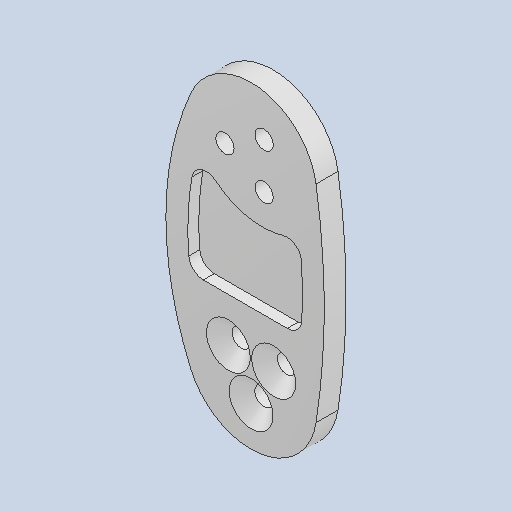
# Autodesk Inventor part: クランク_中間
Saved by Autodesk Inventor 2023 (Build 270158000, 158)
## iProperties
Created: 2022-01-08
Part Number: クランク_中間
Material: Aluminum 2014-T6
Document SubType Name: Modeling
Designer: acps
Density: 2.78927 g/cm^3
Appearance: Satin
Author: acps
Autodesk Inventor part; units mm, degrees
ref_plane "YZ Plane" through (0, 0, 0) normal (1, 0, 0) x (0, 1, 0)
ref_plane "XZ Plane" through (0, 0, 0) normal (0, 1, 0) x (-1, 0, 0)
ref_plane "XY Plane" through (0, 0, 0) normal (0, 0, 1) x (1, 0, 0)
sketch "Sketch2" plane through (0, 0, 0) normal (0, 0, 1) x (1, 0, 0)
  line L0 (-3.5796, 0) -> (-32.4095, 0) construction
  line L1 (-3.5796, 0) -> (-16.3075, 12.7279) construction
  line L2 (-3.5796, 0) -> (-16.3075, -12.7279) construction
  line L3 (-16.3075, 12.7279) -> (-16.3075, -12.7279) construction
  circle A0 centre (-14.5177, 15.8279) radius 1.25
  circle A1 centre (-14.5177, 15.8279) radius 3.1 construction
  circle A2 centre (-19.8871, 12.7279) radius 3.1 construction
  circle A3 centre (-19.8871, 12.7279) radius 1.25
  circle A4 centre (-14.5177, 9.6279) radius 3.1 construction
  circle A5 centre (-14.5177, 9.6279) radius 1.25
  circle A6 centre (-19.4075, -10.9381) radius 1.25
  circle A7 centre (-16.3075, -16.3075) radius 1.25
  circle A8 centre (-13.2075, -10.9381) radius 1.25
  line L4 (-16.3075, 12.7279) -> (-16.3075, -12.7279) construction
  line L5 (-25.3075, 12.7279) -> (-25.3075, -12.7279) construction
  line L6 (-7.3075, -12.7279) -> (-7.3075, 12.7279) construction
  arc A9 (-7.4179, 14.1335) -> (-24.5596, 16.3199) centre (-16.3075, 12.7279) ccw
  arc A10 (-24.5596, -16.3199) -> (-7.4179, -14.1335) centre (-16.3075, -12.7279) ccw
  arc A11 (-24.5596, 16.3199) -> (-24.5596, -16.3199) centre (12.9335, 0) ccw
  arc A12 (-7.4179, -14.1335) -> (-7.4179, 14.1335) centre (-96.8075, 0) ccw
  point P0 (0, 0)
  point P1 (-16.3075, 0)
  point P2 (-16.3075, 0)
  point P3 (-27.9575, 0)
  point P4 (-6.3075, 0)
  dimension "d20" = 18
  dimension "d21" = 18
  dimension "d22" = 90
  dimension "d23" = 2.5
  dimension "d24" = 6.2
  dimension "d25" = 360
  dimension "d26" = 2.5
  dimension "d27" = 360
  dimension "d28" = 6.2
  dimension "d29" = 9
  dimension "d30" = 11.65
  dimension "d31" = 10
  constraints: 18 end point, 13 centre point, 10 point on circle, 9 tangent, 3 coincident, 2 equal length, 2 midpoint, 1 horizontal, 1 horizontal alignment, 1 vertical, 1 vertical alignment, 21 other
  measures "d20" distance of L0.start L1.end
  measures "d21" distance of L0.start L2.end
  measures "d22" angle of L2 L1
  measures "d23" diameter of A0
  measures "d24" diameter of A1
  measures "d26" diameter of A6
  measures "d28" distance of A8.centre A6.centre
  measures "d29" radius of A10
  measures "d30" distance of point (-27.957, 0) point (-16.307, 0)
  measures "d31" distance of point (-6.307, 0) point (-16.307, 0)
extrude "Extrusion1" add sketch "Sketch2" along normal blind 3
chamfer "Chamfer1" distance 1.75 angle 45 3 edges at (-14.4575, -10.9381, 3) (-20.6575, -10.9381, 3) (-17.5575, -16.3075, 3)
sketch "Sketch3" plane through (0, 0, 3) normal (0, 0, 1) x (1, 0, 0)
  circle A0 centre (-14.5177, 9.6279) radius 1.25 projected
  circle A1 centre (-19.8871, 12.7279) radius 1.25 projected
  arc A2 (-24.5596, 16.3199) -> (-24.5596, -16.3199) centre (12.9335, 0) ccw projected
  arc A3 (-7.4179, -14.1335) -> (-7.4179, 14.1335) centre (-96.8075, 0) ccw projected
  circle A4 centre (-19.4075, -10.9381) radius 3 projected
  circle A5 centre (-13.2075, -10.9381) radius 3 projected
  arc A6 (-24.4014, 6.4677) -> (-24.8303, -3.1019) centre (12.9335, 0) ccw
  arc A7 (-9.3592, -3.0069) -> (-9.3967, 3.9499) centre (-96.8075, 0) ccw
  arc A8 (-21.1558, 7.6672) -> (-24.4014, 6.4677) centre (-22.4308, 6.1263) ccw
  arc A9 (-21.1558, 7.6672) -> (-11.959, 5.7783) centre (-14.781, 15.3719) ccw
  arc A10 (-9.3967, 3.9499) -> (-11.959, 5.7783) centre (-11.3947, 3.8596) ccw
  circle A11 centre (-19.8871, 12.7279) radius 1.25 projected
  arc A12 (-20.9971, 12.1531) -> (-14.4605, 8.3792) centre (-14.781, 15.3719) ccw
  arc A13 (-24.8303, -3.1019) -> (-22.837, -4.9381) centre (-22.837, -2.9381) ccw
  line L0 (-19.4075, -7.9381) -> (-13.2075, -7.9381)
  line L1 (-22.837, -4.9381) -> (-11.358, -4.9381)
  arc A14 (-11.358, -4.9381) -> (-9.3592, -3.0069) centre (-11.358, -2.9381) ccw
  point P0 (0, 0)
  dimension "d37" = 3
  dimension "d38" = 3
  dimension "d39" = 2
  dimension "d40" = 3
  dimension "d41" = 2
  dimension "d42" = 7
  dimension "d43" = 2
  dimension "d44" = 2
  dimension "d45" = 3
  constraints: 16 point on circle, 9 tangent, 8 centre point, 4 end point, 2 horizontal, 2 vertical alignment, 1 concentric, 1 parallel, 7 other
  measures "d37" radial gap between concentric circles of A2 A6
  measures "d38" radial gap between concentric circles of A3 A7
  measures "d39" radius of A8
  measures "d40" radial gap between concentric circles of A9 A12
  measures "d41" radius of A10
  measures "d42" radius of A12
  measures "d43" radius of A13
  measures "d44" radius of A14
  measures "d45" distance between parallel lines of L0 L1
extrude "Extrusion2" cut sketch "Sketch3" against normal blind 1.5 contours A8 A9 A10 A7 A14 L1 A13 A6
sketch "sesaku" plane through (0, 0, 3) normal (0, 0, 1) x (1, 0, 0)
  arc A0 (-24.8303, -3.1019) -> (-22.837, -4.9381) centre (-22.837, -2.9381) ccw projected
  arc A1 (-24.4014, 6.4677) -> (-24.8303, -3.1019) centre (12.9335, 0) ccw projected
  arc A2 (-21.1558, 7.6672) -> (-24.4014, 6.4677) centre (-22.4308, 6.1263) ccw projected
  arc A3 (-21.1558, 7.6672) -> (-11.959, 5.7783) centre (-14.781, 15.3719) ccw projected
  arc A4 (-9.3967, 3.9499) -> (-11.959, 5.7783) centre (-11.3947, 3.8596) ccw projected
  arc A5 (-9.3592, -3.0069) -> (-9.3967, 3.9499) centre (-96.8075, 0) ccw projected
  arc A6 (-11.358, -4.9381) -> (-9.3592, -3.0069) centre (-11.358, -2.9381) ccw projected
  line L0 (-11.358, -4.9381) -> (-22.837, -4.9381) projected
  circle A7 centre (-19.4075, -10.9381) radius 3 projected
  circle A8 centre (-14.5177, 15.8279) radius 1.25 projected
  circle A9 centre (-14.5177, 9.6279) radius 1.25 projected
  circle A10 centre (-19.8871, 12.7279) radius 1.25 projected
  arc A11 (-24.5596, 16.3199) -> (-24.5596, -16.3199) centre (12.9335, 0) ccw projected
  arc A12 (-24.5596, -16.3199) -> (-7.4179, -14.1335) centre (-16.3075, -12.7279) ccw projected
  arc A13 (-7.4179, -14.1335) -> (-7.4179, 14.1335) centre (-96.8075, 0) ccw projected
  arc A14 (-7.4179, 14.1335) -> (-24.5596, 16.3199) centre (-16.3075, 12.7279) ccw projected
  circle A15 centre (-13.2075, -10.9381) radius 3 projected
  circle A16 centre (-16.3075, -16.3075) radius 3 projected
  circle A17 centre (-19.4075, -10.9381) radius 1.25 projected
  circle A18 centre (-19.4075, -10.9381) radius 3 projected
  circle A19 centre (-13.2075, -10.9381) radius 1.25 projected
  circle A20 centre (-16.3075, -16.3075) radius 1.25 projected
  point P0 (0, 0)
body "Solid1"
